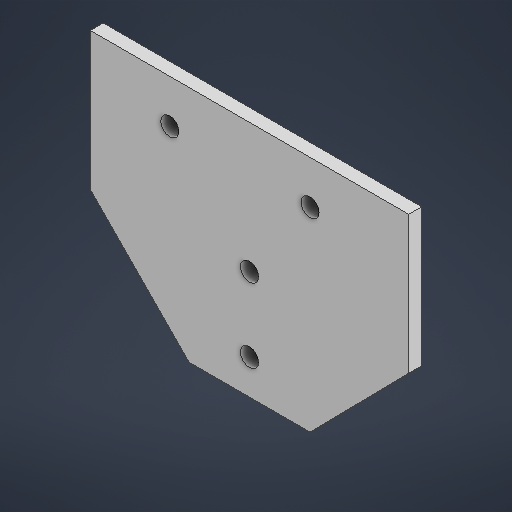
# Autodesk Inventor part: трапеция для профиля
Saved by Autodesk Inventor 2025 (Build 290162000, 162)
## iProperties
Created: 2024-10-09
Part Number: трапеция для профиля
Material: Типовые
Document SubType Name: Modeling
Designer: Phantom
Density: 1 g/cm^3
Appearance: По умолчанию
Author: Phantom
Autodesk Inventor part; units mm, degrees
ref_plane "YZ Plane" through (0, 0, 0) normal (1, 0, 0) x (0, 1, 0)
ref_plane "XZ Plane" through (0, 0, 0) normal (0, 1, 0) x (-1, 0, 0)
ref_plane "XY Plane" through (0, 0, 0) normal (0, 0, 1) x (1, 0, 0)
sketch "Эскиз1" plane through (0, 0, 0) normal (0, 0, 1) x (1, 0, 0)
  line L0 (19.4917, 4.2381) -> (56.3509, 4.2381)
  line L1 (19.4917, -27.8221) -> (19.4917, 4.2381)
  line L2 (23.9917, -27.8221) -> (19.4917, -27.8221)
  line L3 (23.9917, -27.8221) -> (53.5066, 2.1779)
  line L4 (53.5066, 2.1779) -> (57.0345, 2.1779)
  line L5 (57.0345, 2.1779) -> (56.3509, 4.2381)
  line L6 (27.9917, 2.1779) -> (44.5248, 2.1779)
  arc A0 (45.9505, -1.2247) -> (44.5248, 2.1779) centre (44.5248, 0.1779) ccw
  line L7 (45.9505, -1.2247) -> (27.4174, -20.0624)
  arc A1 (23.9917, -18.6598) -> (27.4174, -20.0624) centre (25.9917, -18.6598) ccw
  line L8 (23.9917, -18.6598) -> (23.9917, -1.8221)
  arc A2 (27.9917, 2.1779) -> (23.9917, -1.8221) centre (27.9917, -1.8221) ccw
  line L9 (-39.3572, 4.2381) -> (0.4917, 4.2381)
  arc A3 (-36.4955, 2.1779) -> (-39.3572, 4.2381) centre (-50.0058, -13.5712) ccw
  line L10 (-36.4955, 2.1779) -> (-33.5231, 2.1779)
  line L11 (-33.5231, 2.1779) -> (-4.0083, -27.8221)
  line L12 (-4.0083, -27.8221) -> (0.4917, -27.8221)
  line L13 (0.4917, 4.2381) -> (0.4917, -27.8221)
  line L14 (-24.5413, 2.1779) -> (-8.0083, 2.1779)
  arc A4 (-4.0083, -1.8221) -> (-8.0083, 2.1779) centre (-8.0083, -1.8221) ccw
  line L15 (-4.0083, -1.8221) -> (-4.0083, -18.6598)
  arc A5 (-7.434, -20.0624) -> (-4.0083, -18.6598) centre (-6.0083, -18.6598) ccw
  line L16 (-7.434, -20.0624) -> (-25.967, -1.2247)
  arc A6 (-24.5413, 2.1779) -> (-25.967, -1.2247) centre (-24.5413, 0.1779) ccw
  line L17 (19.4917, -27.8221) -> (0.4917, -27.8221)
  line L18 (46.796, 27.1824) -> (46.796, -12.8221)
  line L19 (9.9917, -27.8221) -> (9.9917, 27.1824)
  line L20 (74.6897, 27.1824) -> (-75.7558, 27.1824)
  line L21 (46.796, 27.1824) -> (9.9917, 27.1824)
  line L22 (-26.8126, 27.1824) -> (9.9917, 27.1824)
  line L23 (-26.8126, 27.1824) -> (-26.8126, -10.6435)
  arc A7 (-53.8558, 14.0224) -> (-53.8558, 18.2224) centre (-53.8558, 16.1224) ccw
  line L24 (-53.8558, 16.1224) -> (53.5066, 16.1824)
  line L25 (73.7569, 16.1824) -> (46.796, 16.1824)
  point P0 (0, 0)
  point P1 (46.796, -4.6429)
  point P2 (-26.8126, -4.6429)
  constraints: 52 end point, 16 point on circle, 8 centre point, 3 perpendicular, 2 point on line, 2 vertical, 1 midpoint, 1 symmetric about line
extrude "Выдавливание1" add sketch "Эскиз1" along normal blind 3 contours L1 L17 L19 L24 L18 L0 | L0 L18 L3 L2 L1 | L24 L19 L20 L18 | L17 L13 L9 L23 L24 L19 | L24 L23 L20 L19 | L12 L11 L23 L9 L13 | L6 A0 L7 A1 L8 A2 | L14 A4 L15 A5 L16 A6
sketch "Эскиз2" plane through (0, 0, 0) normal (0, 0, -1) x (-1, 0, 0)
  line L0 (4.0083, -27.8221) -> (-23.9917, -27.8221) projected
  line L1 (-9.9917, -27.8221) -> (-9.9917, 27.1824)
  line L2 (-46.796, 27.1824) -> (26.8126, 27.1824) projected
  line L3 (26.8126, 27.1824) -> (26.8126, -4.6429) projected
  line L4 (26.8126, 11.2697) -> (-46.796, 11.2697)
  line L5 (-46.796, -4.6429) -> (-46.796, 27.1824) projected
  line L6 (4.0083, -27.8221) -> (4.0083, 40.673)
  line L7 (-23.9917, -27.8221) -> (-23.9917, 46.5854)
  line L8 (-9.9917, -27.8221) -> (-9.9917, -19.8221)
  circle A0 centre (-9.9917, -19.8221) radius 2.1
  line L9 (-9.9917, -17.7221) -> (-9.9917, -2.7221)
  circle A1 centre (-9.9917, -2.7221) radius 2.1
  line L10 (4.0083, 13.3697) -> (4.0083, 17.3697)
  line L11 (4.0083, 27.1824) -> (4.0083, 16.1824)
  line L12 (-23.9917, 27.1824) -> (-23.9917, 17.1824)
  circle A2 centre (-23.9917, 17.1824) radius 2.1
  line L13 (4.0083, 18.2824) -> (4.0083, 22.2824)
  line L14 (4.0083, 22.2824) -> (29.571, 22.2824)
  line L15 (29.571, 22.2824) -> (-56.1898, 22.2824)
  line L16 (-23.9917, 22.2824) -> (-28.4167, 22.2824)
  line L17 (-28.4167, 22.2824) -> (-28.4167, 3.0492)
  line L18 (4.0083, 22.2824) -> (8.4333, 22.2824)
  line L19 (8.4333, 22.2824) -> (8.4333, 2.2797)
  circle A3 centre (8.4333, 17.1824) radius 2.1
  point P0 (0, 0)
  point P1 (26.8126, 22.2824)
  point P2 (-46.796, 22.2824)
  point P3 (-28.4167, 17.1824)
  dimension "d5" = 4.2
  dimension "d4" = 8
  dimension "d6" = 15
  dimension "d7" = 4.2
  dimension "d12" = 10
  dimension "d19" = 4.425
  dimension "d20" = 4.425
  constraints: 32 end point, 20 point on line, 4 midpoint, 3 centre point, 3 perpendicular, 2 coincident, 2 vertical, 1 vertical alignment, 2 other
  measures "d4" distance of L1.start L8.end
  measures "d6" distance of L9.start L9.end
  measures "d7" diameter of A1
  measures "d12" distance of L12.start L12.end
  measures "d19" distance of L16.start L16.end
  measures "d20" distance of L13.end L18.end
extrude "Выдавливание2" cut sketch "Эскиз2" against normal blind 3 contours A0 L1 | L1 A0 | A3 L19 | L19 A3 | A1 L1 | L1 A1 | A2 L7 | L7 A2
